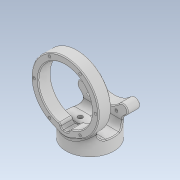
# Autodesk Inventor part: hip_link
Saved by Autodesk Inventor 2020 (Build 240168000, 168)
## iProperties
Created: 2020-12-22
Part Number: hip_link
Material: Generic
Document SubType Name: Modeling
Designer: DELL
Density: 1 g/cm^3
Appearance: Default
Author: DELL
Autodesk Inventor part; units mm, degrees
ref_plane "YZ Plane" through (0, 0, 0) normal (1, 0, 0) x (0, 1, 0)
ref_plane "XZ Plane" through (0, 0, 0) normal (0, 1, 0) x (-1, 0, 0)
sketch "Sketch1" plane through (0, 0, 0) normal (0, 1, 0) x (-1, 0, 0)
  circle A0 centre (0, 0) radius 11.5 construction
  circle A1 centre (11.5, 0) radius 1.65
  circle A2 centre (-5.75, -9.9593) radius 1.65
  circle A3 centre (-5.75, 9.9593) radius 1.65
  line L0 (0, 0) -> (11.5, 0) construction
  line L1 (0, 0) -> (-5.75, 9.9593) construction
  line L2 (0, 0) -> (-5.75, -9.9593) construction
  circle A4 centre (0, 0) radius 9.715 construction
  circle A5 centre (4.8575, 8.4134) radius 2
  circle A6 centre (4.8575, -8.4134) radius 2
  circle A7 centre (-9.715, 0) radius 2
  line L3 (4.8575, 8.4134) -> (0, 0) construction
  line L4 (0, 0) -> (4.8575, -8.4134) construction
  line L5 (0, 0) -> (-9.715, 0) construction
  circle A8 centre (0, 0) radius 17.5 construction
  circle A9 centre (0, 0) radius 28
  circle A10 centre (11.5, 0) radius 2.75
  circle A11 centre (-5.75, 9.9593) radius 2.75
  circle A12 centre (-5.75, -9.9593) radius 2.75
  line L6 (23.9531, 14.5) -> (-23.9531, 14.5)
  line L7 (23.9531, -14.5) -> (-23.9531, -14.5)
  dimension "d0" = 23
  dimension "d1" = 120
  dimension "d2" = 120
  dimension "d3" = 3.3
  dimension "d4" = 19.43
  dimension "d5" = 4
  dimension "d6" = 120
  dimension "d7" = 120
  dimension "d8" = 35
  dimension "d9" = 56
  dimension "d12" = 5.5
  dimension "d34" = 29
  constraints: 16 end point, 13 centre point, 10 point on circle, 7 coincident, 6 equal radius, 3 horizontal, 1 parallel, 1 other
  measures "d0" diameter of A0
  measures "d1" angle of L0 L1
  measures "d2" angle of L0 L2
  measures "d3" diameter of A1
  measures "d4" diameter of A4
  measures "d5" diameter of A5
  measures "d6" angle of L5 L3
  measures "d7" angle of L5 L4
  measures "d8" diameter of A8
  measures "d9" diameter of A9
  measures "d12" diameter of A11
  measures "d34" distance between parallel lines of L7 L6
extrude "Extrusion1" add sketch "Sketch1" against normal blind 15 contours A9 L7 L6 | L6 A9 | A9 L7 | A10 | A11 | A12
extrude "Extrusion3" cut sketch "Sketch1" against normal blind 5 contours A10 | A11 | A12
sketch "Sketch2" plane through (0, 0, 0) normal (0, 0, 1) x (1, 0, 0)
  circle A0 centre (0, 42) radius 36
  circle A1 centre (0, 42) radius 33 construction
  circle A2 centre (-18, 73.1769) radius 1.5
  circle A3 centre (18, 73.1769) radius 1.5
  line L0 (-36, 42) -> (36, 42) construction
  circle A4 centre (-36, 42) radius 1.5
  circle A5 centre (36, 42) radius 1.5
  circle A6 centre (-18, 10.8231) radius 1.5
  circle A7 centre (18, 10.8231) radius 1.5
  line L1 (-18, 73.1769) -> (0, 42) construction
  line L2 (0, 0) -> (0, 78) construction
  line L3 (28, 0) -> (-28, 0) construction
  circle A8 centre (0, 42) radius 39.5 construction
  circle A9 centre (-33, 42) radius 1.65
  circle A10 centre (33, 42) radius 1.65
  circle A11 centre (0, 42) radius 39.5
  circle A12 centre (0, 42) radius 28
  arc A13 (27.9307, 14.0693) -> (19.799, 22.201) centre (23.8649, 18.1351) ccw
  arc A14 (-19.799, 22.201) -> (-27.9307, 14.0693) centre (-23.8649, 18.1351) ccw
  circle A15 centre (16.5, 13.4212) radius 1.65
  circle A16 centre (-16.5, 13.4212) radius 1.65
  line L4 (0, 42) -> (16.5, 13.4212) construction
  circle A17 centre (0, 42) radius 31.5
  line L5 (0, 42) -> (23.8649, 18.1351) construction
  line L6 (5, 10.8994) -> (5, 2.8177)
  line L7 (-5, 10.8994) -> (-5, 2.8177)
  point P0 (34.5788, 41.5204)
  point P1 (34.5788, 42.4796)
  point P2 (31.4928, 41.3285)
  point P3 (16.328, 15.0622)
  point P4 (15.1648, 14.3906)
  point P5 (-15.1648, 14.3906)
  point P6 (-16.328, 15.0622)
  point P7 (-31.4928, 41.3285)
  point P8 (-31.4928, 42.6715)
  point P9 (31.4928, 42.6715)
  point P10 (5, 6.3489)
  point P11 (-5, 6.3489)
  dimension "d17" = 72
  dimension "d18" = 66
  dimension "d19" = 3
  dimension "d20" = 60
  dimension "d21" = 79
  dimension "d22" = 42
  dimension "d30" = 56
  dimension "d31" = 3.3
  dimension "d32" = 60
  dimension "d33" = 63
  dimension "d37" = 45
  dimension "d44" = 10
  constraints: 17 centre point, 16 point on circle, 14 end point, 9 equal radius, 7 coincident, 4 symmetric about line, 4 tangent, 2 point on line, 1 horizontal, 1 midpoint, 1 parallel, 1 perpendicular, 1 vertical, 11 other
  measures "d18" diameter of A1
  measures "d19" diameter of A2
  measures "d20" angle of L0 L1
  measures "d21" diameter of A8
  measures "d22" distance from line of L3 L1.end
  measures "d30" diameter of A12
  measures "d31" diameter of A10
  measures "d32" angle of L0 L4
  measures "d33" diameter of A17
  measures "d37" angle of L2 L5
  measures "d44" distance between parallel lines of L7 L6
ref_plane "Work Plane1" through (0, 0, 14.5) normal (0, 0, 1) x (1, 0, 0)
ref_plane "Work Plane2" through (0, 0, -14.5) normal (0, 0, 1) x (1, 0, 0)
extrude "Extrusion4" add sketch "Sketch2" along normal blind 15 from surface at 14.5 contours A5 A10 A17 A9 A4 A0 A2 A3 | A0 A3 A2 A4 A14 A11 A13 A5 | A0 A13 A17 A10 A5 | A5 A10 A17 | A13 A11 L6 A0 A7 | A0 A7 A15 A17 A13 | A17 A9 A4 | A0 L6 A17 A15 A7 | A7 A15 A17 | A11 L7 A0 L6 | A17 A14 A0 A4 A9 | A11 A14 A0 A6 L7 | A17 A16 A6 A0 A14 | A0 A6 A16 A17 L7 | A17 A16 A6
extrude "Extrusion5" add sketch "Sketch2" against normal blind 15 from surface at -14.5 contours A13 A11 L6 A0 A7 | A0 A7 A15 A17 A13 | A7 A0 | A0 A7 A15 | A17 A15 A16 A14 A12 A13 | A0 L6 A17 A15 A7 | A11 L7 A0 L6 | A0 L7 A17 L6 | A11 A14 A0 A6 L7 | A17 A16 A6 A0 A14 | A0 A6 A16 A17 L7 | A6 A0 | A0 A6 A16
extrude "Extrusion6" add sketch "Sketch1" along normal up to surface contours L6 A9 | A9 L7 round surface about axis through (0, 42, 0) along (0, 0, 1) radius 39.5 far side no
fillet "Fillet1" radius 5 2 edges at (-0.0007, 2.5, 28) (-0.0007, 2.5, -28)
fillet "Fillet2" radius 7 2 edges at (0, 0, 14.5) (0, 0, -14.5)
fillet "Fillet3" radius 3 6 edges at (5, 6.3489, 14.4848) (5, 6.3489, 22) (-5, 6.3489, 14.4848) (-5, 6.3489, 22) (-5, 10.8994, 22) (5, 10.8994, 22)
fillet "Fillet6" radius 1 55 edges at (33.4757, 21.0327, 14.5) (-33.4757, 21.0327, 14.5) (39.1207, 36.5395, 14.5) (-5.4605, 81.1207, 14.5) (-24.6371, 10.35, 14.5) (-23.9531, 7.3005, 14.5) (-24.9348, 2.3563, 12.738) (-27.743, 0, 3.7847) (-27.743, 0, -3.7847) (-24.9407, 2.3433, -12.7264) (-23.9531, 7.3005, -14.5) (-24.6371, 10.35, -14.5) (-27.1326, 13.2934, -14.5) (-27.9307, 22.201, -14.5) (0, 14, -14.5) (27.9307, 22.201, -14.5) (27.1326, 13.2934, -14.5) (24.6371, 10.35, -14.5) (23.9531, 7.3005, -14.5) (24.9407, 2.3433, -12.7264) (28, 0, 0) (24.9348, 2.3563, 12.738) (23.9531, 7.3005, 14.5) (24.6371, 10.35, 14.5) (21.0522, 8.5776, -29.5) (0, 1.0707, -29.5) (-21.0522, 8.5776, -29.5) (-27.9307, 22.201, -29.5) (0, 14, -29.5) (27.9307, 22.201, -29.5) (11.4196, 4.1154, 29.5) (0, 1.0707, 29.5) (-11.4196, 4.1154, 29.5) (28.4221, 14.5695, 29.5) (39.0466, 36.0327, 29.5) (-5.9673, 81.0466, 29.5) (-28.4221, 14.5695, 29.5) (-4.0739, 6.8929, 29.5) (0, 6, 29.5) (4.0739, 6.8929, 29.5) (8.5243, 11.6753, 29.5) (26.7714, 25.4006, 29.5) (0, 73.5, 29.5) (-26.7714, 25.4006, 29.5) (-8.5243, 11.6753, 29.5) (-4.7256, 7.8072, 14.5) (-3.2339, 6.3261, 14.4675) (0, 6, 14.4282) (3.2339, 6.3261, 14.4675) (4.7256, 7.8072, 14.5) (26.479, 24.938, 14.5) (8.462, 11.6579, 14.5) (-8.462, 11.6579, 14.5) (-26.479, 24.938, 14.5) (0, 73.5, 14.5)
body "Solid1"
